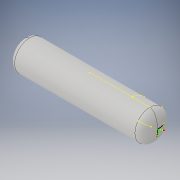
# Autodesk Inventor part: ModeloVaso
Saved by Autodesk Inventor 2019 (Build 230136000, 136)
## iProperties
Created: 2018-09-09
Part Number: ModeloVaso
Material: Generic
Document SubType Name: Modeling
Designer: leona
Density: 1 g/cm^3
Appearance: Default
Author: leona
Autodesk Inventor part; units mm, degrees
ref_plane "XY Plane" through (0, 0, 0) normal (0, 0, 1) x (1, 0, 0)
sketch "Sketch1" plane through (0, 0, 0) normal (0, 0, 1) x (1, 0, 0)
  line L0 (0, 50) -> (0, 0) construction
  line L1 (0, 0) -> (200, 0)
  line L2 (0, 50) -> (200, 50)
  ellipse E0 centre (200, 0) end of major axis (200, 50) minor radius 25 (225, 0) -> (200, 50) ccw
  line L3 (200, 0) -> (225, 0)
  line L4 (0, 50) -> (0, 0)
  line L5 (225, 0) -> (0, 0)
  dimension "d2" = 25
  dimension "d0" = 50
  dimension "d1" = 200
  constraints: 12 end point, 3 horizontal, 2 perpendicular, 1 coincident, 1 collinear, 1 point on line, 1 vertical, 4 other
  measures "d0" distance of L0.start L0.end
  measures "d1" distance of L0.end L1.end
revolve "Revolution1" add sketch "Sketch1" angle 360 about axis through (0, 0, 0) along (1, 0, 0)
mirror "Mirror1" about plane through (0, 50, 0) normal (-1, 0, 0) of "Revolution1"
ref_plane "Work Plane1" through (100, -50, 0) normal (0, 1, 0) x (-1, 0, 0)
sketch "Sketch2" plane through (100, -50, 0) normal (0, 1, 0) x (-1, 0, 0)
  line L0 (-125, 0) -> (-100, 0) projected
  line L1 (-100, 0) -> (100, 0)
  line L2 (-41.797, 0) -> (-41.797, -39.5982)
  line L3 (-41.797, -39.5982) -> (-100, -39.5982)
  line L4 (-100, 50) -> (-100, -50) projected
  constraints: 6 end point, 2 point on line, 1 horizontal, 1 perpendicular, 1 vertical
sketch3d "3D Sketch1"
ref_plane "Work Plane2" through (200, -30.5284, -39.5982) normal (0, -0.6105678, -0.791964) x (1, 0, 0)
sketch "Sketch3" plane through (200, -30.5284, -39.5982) normal (0, -0.6105678, -0.791964) x (1, 0, 0)
  line L0 (0, -50) -> (0, 50) projected
  line L1 (0, 0) -> (22, 0)
  point P0 (-200, 0)
  point P1 (0, -39.5982)
  dimension "d5" = 22
  constraints: 2 end point, 1 horizontal, 1 midpoint
  measures "d5" distance of L1.start L1.end
sketch3d "3D Sketch2"
ref_plane "Work Plane3" through (225, 0, 0) normal (1, 0, 0) x (0, 1, 0)
sketch "Sketch4" plane through (225, 0, 0) normal (1, 0, 0) x (0, 1, 0)
  line L0 (0, 0) -> (0, -20)
  line L1 (0, -20) -> (-1, -20)
  line L2 (1, -20) -> (0, -20)
  line L3 (1, -20) -> (0, -25)
  line L4 (0, -25) -> (-1, -20)
  line L5 (-20, 0) -> (-20, 1)
  line L6 (-20, -1) -> (-20, 0)
  line L7 (-20, -1) -> (-25, 0)
  line L8 (-25, 0) -> (-20, 1)
  line L9 (0, 0) -> (-20, 0)
  line L10 (0, 0) -> (50, 0) projected
  line L11 (0, 0) -> (-14.5002, -18.8081)
  arc A0 (-13.3135, 0) -> (-8.1288, -10.5438) centre (0, 0) ccw
  dimension "d6" = 1
  dimension "d13" = 5
  dimension "d14" = 20
  dimension "d17" = 90
  constraints: 22 end point, 4 point on line, 3 coincident, 2 collinear, 2 point on circle, 1 centre point, 1 perpendicular, 1 vertical, 10 other
  measures "d6" distance of L0.end L1.end
  measures "d13" vertical distance of L2.start L3.end
  measures "d14" distance of L0.start L0.end
sketch3d "3D Sketch3"
body "Solid1"
